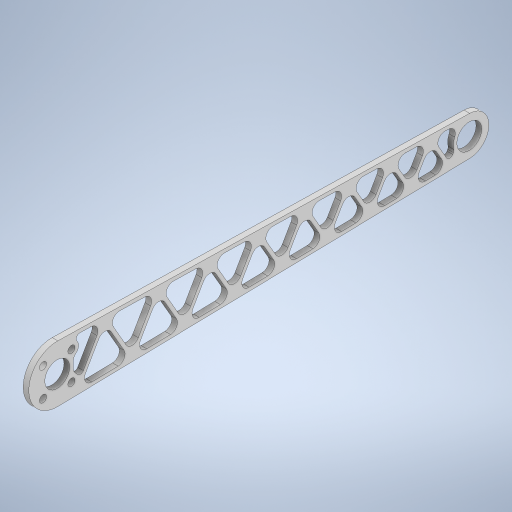
# Autodesk Inventor part: arm
Saved by Autodesk Inventor 2023 (Build 270158000, 158)
## iProperties
Created: 2022-09-10
Part Number: arm
Material: Generic
Document SubType Name: Modeling
Designer: deli
Density: 1 g/cm^3
Appearance: Default
Mass: 20.635 g
Surface Area: 151.802 cm^2
Volume: 20.635 cm^3
Author: deli
Autodesk Inventor part; units mm, degrees
ref_plane "YZ Plane" through (0, 0, 0) normal (1, 0, 0) x (0, 1, 0)
ref_plane "XZ Plane" through (0, 0, 0) normal (0, 1, 0) x (-1, 0, 0)
ref_plane "XY Plane" through (0, 0, 0) normal (0, 0, 1) x (1, 0, 0)
sketch "Sketch1" plane through (0, 0, 0) normal (1, 0, 0) x (0, 1, 0)
  circle A0 centre (62.068154, -4.109119) radius 2
  circle A1 centre (62.068154, -20.109119) radius 2
  circle A2 centre (46.068154, -20.109119) radius 2
  circle A3 centre (46.068154, -4.109119) radius 2
  line L0 (62.068154, -4.109119) -> (62.068154, -20.109119) construction
  line L1 (62.068154, -20.109119) -> (46.068154, -20.109119) construction
  line L2 (46.068154, -20.109119) -> (46.068154, -4.109119) construction
  line L3 (46.068154, -4.109119) -> (62.068154, -4.109119) construction
  circle A4 centre (54.068154, -12.109119) radius 7
  line L4 (62.068154, -4.109119) -> (46.068154, -20.109119) construction
  line L5 (62.068154, -20.109119) -> (46.068154, -4.109119) construction
  arc A5 (70.064438, -12.453946) -> (38.071871, -12.453946) centre (54.068154, -12.109119) ccw
  circle A6 centre (54.068154, -244.109119) radius 7
  line L6 (54.068154, -12.109119) -> (54.068154, -244.109119) construction
  arc A7 (43.070709, -244.346188) -> (65.065599, -244.346188) centre (54.068154, -244.109119) ccw
  line L7 (70.064438, -12.453946) -> (65.065599, -244.346188)
  line L8 (43.070709, -244.346188) -> (38.071871, -12.453946)
  line L9 (46.068154, -20.109119) -> (40.450729, -23.352341) construction
  line L10 (40.450729, -23.352341) -> (67.492484, -38.964905) construction
  line L11 (67.492484, -38.964905) -> (40.97387, -54.275434) construction
  line L12 (40.97387, -54.275434) -> (66.840508, -69.209545) construction
  line L13 (66.840508, -69.209545) -> (41.609816, -83.776492) construction
  line L14 (41.609816, -83.776492) -> (66.220197, -97.985302) construction
  line L15 (42.214877, -111.84478) -> (66.220197, -97.985302) construction
  line L16 (42.214877, -111.84478) -> (65.630012, -125.363515) construction
  line L17 (65.630012, -125.363515) -> (42.790551, -138.549883) construction
  line L18 (42.790551, -138.549883) -> (65.068491, -151.412058) construction
  line L19 (65.068491, -151.412058) -> (43.338268, -163.958008) construction
  line L20 (43.338268, -163.958008) -> (64.534241, -176.195509) construction
  line L21 (64.534241, -176.195509) -> (43.859383, -188.132144) construction
  line L22 (43.859383, -188.132144) -> (64.025937, -199.775309) construction
  line L23 (64.025937, -199.775309) -> (44.355189, -211.132221) construction
  line L24 (44.355189, -211.132221) -> (63.54232, -222.209916) construction
  line L25 (63.54232, -222.209916) -> (44.826916, -233.01526) construction
  line L26 (44.826916, -233.01526) -> (50.027004, -236.017532) construction
  line L27 (44.802331, -231.874754) -> (61.54232, -222.209916)
  line L28 (61.54232, -222.209916) -> (44.380395, -212.301473)
  line L29 (44.330604, -209.991715) -> (62.025937, -199.775309)
  line L30 (62.025937, -199.775309) -> (43.884588, -189.301396)
  line L31 (43.834797, -186.991637) -> (62.534241, -176.195509)
  line L32 (62.534241, -176.195509) -> (43.363473, -165.127261)
  line L33 (43.313682, -162.817502) -> (63.068491, -151.412058)
  line L34 (63.068491, -151.412058) -> (42.815757, -139.719136)
  line L35 (42.765966, -137.409377) -> (63.630012, -125.363515)
  line L36 (63.630012, -125.363515) -> (42.240082, -113.014033)
  line L37 (42.190291, -110.704274) -> (64.220197, -97.985302)
  line L38 (64.220197, -97.985302) -> (41.635021, -84.945744)
  line L39 (41.585231, -82.635985) -> (64.840508, -69.209545)
  line L40 (64.840508, -69.209545) -> (40.999075, -55.444687)
  line L41 (40.949284, -53.134928) -> (65.492484, -38.964905)
  line L42 (65.492484, -38.964905) -> (40.330666, -24.437723)
  line L43 (50.511319, -235.142451) -> (49.826916, -234.747311)
  line L44 (49.826916, -231.283209) -> (63.517115, -223.379169)
  line L45 (63.566906, -221.06941) -> (46.355189, -211.132221)
  line L46 (46.355189, -211.132221) -> (64.000732, -200.944562)
  line L47 (64.050523, -198.634803) -> (45.859383, -188.132144)
  line L48 (45.859383, -188.132144) -> (64.509035, -177.364762)
  line L49 (64.558826, -175.055003) -> (45.338268, -163.958008)
  line L50 (45.338268, -163.958008) -> (65.043286, -152.581311)
  line L51 (65.093076, -150.271552) -> (44.790551, -138.549883)
  line L52 (44.790551, -138.549883) -> (65.604807, -126.532767)
  line L53 (65.654598, -124.223009) -> (44.214877, -111.84478)
  line L54 (44.214877, -111.84478) -> (66.194992, -99.154554)
  line L55 (66.244783, -96.844796) -> (43.609816, -83.776492)
  line L56 (43.609816, -83.776492) -> (66.815303, -70.378797)
  line L57 (66.865094, -68.069039) -> (42.97387, -54.275434)
  line L58 (42.97387, -54.275434) -> (67.467279, -40.134158)
  line L59 (67.517069, -37.824399) -> (48.435104, -26.807421)
  arc A8 (48.312787, -23.419953) -> (49.941138, -21.109119) centre (46.068154, -20.109119) ccw
  arc A9 (63.066064, -244.303084) -> (51.976198, -235.355621) centre (54.068154, -244.109119) ccw
  arc A10 (67.796689, -24.853051) -> (64.554735, -23.242658) centre (65.797154, -24.809948) ccw
  line L60 (63.066064, -244.303084) -> (67.796689, -24.853051)
  arc A11 (58.194893, -21.109119) -> (64.554735, -23.242658) centre (62.068154, -20.109119) ccw
  line L61 (58.194893, -21.109119) -> (49.941138, -21.109119)
  line L62 (40.330666, -24.437723) -> (44.854331, -234.286992)
  arc A12 (48.312787, -23.419953) -> (48.435104, -26.807421) centre (49.435104, -25.07537) ccw
  arc A13 (49.826916, -231.283209) -> (49.826916, -234.747311) centre (50.826916, -233.01526) ccw
  arc A14 (50.511319, -235.142451) -> (51.976198, -235.355621) centre (51.511319, -233.4104) ccw
  point P0 (0, 0)
  dimension "d0" = 4
  dimension "d1" = 4
  dimension "d2" = 4
  dimension "d3" = 4
  dimension "d4" = 16
  dimension "d5" = 16
  dimension "d6" = 14
  dimension "d7" = 32
  dimension "d8" = 14
  dimension "d9" = 232
  dimension "d10" = 4
  dimension "d29" = 120
  dimension "d30" = 60
  dimension "d31" = 60
  dimension "d33" = 1
  dimension "d34" = 1
  dimension "d35" = 4
  dimension "d37" = 1
  dimension "d40" = 4
  dimension "d41" = 2
  dimension "d44" = 4
  dimension "d45" = 4
  dimension "d46" = 1
  dimension "d48" = 1
  dimension "d49" = 1
  dimension "d50" = 1
  dimension "d51" = 1
  dimension "d52" = 1
  dimension "d53" = 1
  dimension "d54" = 1
  dimension "d55" = 1
  dimension "d56" = 1
  dimension "d57" = 1
  dimension "d58" = 1
  dimension "d59" = 1
  dimension "d60" = 1
  dimension "d61" = 1
  dimension "d62" = 1
  dimension "d63" = 1
  dimension "d64" = 1
  dimension "d65" = 1
  dimension "d66" = 1
  dimension "d67" = 1
  dimension "d68" = 1
  dimension "d69" = 1
  dimension "d70" = 1
  dimension "d71" = 1
  dimension "d72" = 1
  dimension "d73" = 1
  dimension "d74" = 1
  dimension "d75" = 1
  dimension "d76" = 1
  dimension "d77" = 1
  dimension "d79" = 2
  dimension "d80" = 2
  constraints: 122 end point, 46 parallel, 18 point on circle, 15 centre point, 10 tangent, 3 coincident, 3 perpendicular, 2 vertical, 1 horizontal, 1 midpoint, 57 other
  measures "d0" diameter of A0
  measures "d1" diameter of A3
  measures "d2" diameter of A2
  measures "d3" diameter of A1
  measures "d4" distance of L0.start L0.end
  measures "d5" distance of L2.end L0.start
  measures "d6" diameter of A4
  measures "d7" diameter of A5
  measures "d8" diameter of A6
  measures "d9" distance of L6.start L6.end
  measures "d10" radial gap between concentric circles of A7 A6
  measures "d29" angle of L2 L9
  measures "d30" angle of L10 L9
  measures "d31" angle of L11 L10
  measures "d33" distance between parallel lines of L10 L42
  measures "d34" distance between parallel lines of L10 L59
  measures "d35" diameter of A10
  measures "d37" distance between parallel lines of L61 L1
  measures "d40" diameter of A12
  measures "d41" radial gap between concentric circles of A2 A8
  measures "d44" diameter of A13
  measures "d45" diameter of A14
  measures "d46" distance between parallel lines of L26 L43
  measures "d48" distance between parallel lines of L27 L25
  measures "d49" distance between parallel lines of L44 L25
  measures "d50" distance between parallel lines of L24 L45
  measures "d51" distance between parallel lines of L28 L24
  measures "d52" distance between parallel lines of L23 L46
  measures "d53" distance between parallel lines of L23 L29
  measures "d54" distance between parallel lines of L22 L47
  measures "d55" distance between parallel lines of L30 L22
  measures "d56" distance between parallel lines of L48 L21
  measures "d57" distance between parallel lines of L21 L31
  measures "d58" distance between parallel lines of L20 L49
  measures "d59" distance between parallel lines of L32 L20
  measures "d60" distance between parallel lines of L50 L19
  measures "d61" distance between parallel lines of L19 L33
  measures "d62" distance between parallel lines of L34 L18
  measures "d63" distance between parallel lines of L18 L51
  measures "d64" distance between parallel lines of L52 L17
  measures "d65" distance between parallel lines of L17 L35
  measures "d66" distance between parallel lines of L36 L16
  measures "d67" distance between parallel lines of L16 L53
  measures "d68" distance between parallel lines of L54 L15
  measures "d69" distance between parallel lines of L15 L37
  measures "d70" distance between parallel lines of L38 L14
  measures "d71" distance between parallel lines of L14 L55
  measures "d72" distance between parallel lines of L56 L13
  measures "d73" distance between parallel lines of L13 L39
  measures "d74" distance between parallel lines of L40 L12
  measures "d75" distance between parallel lines of L12 L57
  measures "d76" distance between parallel lines of L11 L58
  measures "d77" distance between parallel lines of L11 L41
extrude "Extrusion1" add sketch "Sketch1" along normal blind 3.175
fillet "Fillet1" radius 4 50 edges at (1.5875, 49.9411, -21.1091) (1.5875, 67.5171, -37.8244) (1.5875, 65.4925, -38.9649) (1.5875, 67.4673, -40.1342) (1.5875, 42.9739, -54.2754) (1.5875, 40.9493, -53.1349) (1.5875, 40.3307, -24.4377) (1.5875, 58.1949, -21.1091) (1.5875, 66.8651, -68.069) (1.5875, 66.8153, -70.3788) (1.5875, 64.8405, -69.2095) (1.5875, 40.9991, -55.4447) (1.5875, 41.5852, -82.636) (1.5875, 43.6098, -83.7765) (1.5875, 41.635, -84.9457) (1.5875, 66.2448, -96.8448) (1.5875, 64.2202, -97.9853) (1.5875, 66.195, -99.1546) (1.5875, 42.1903, -110.7043) (1.5875, 44.2149, -111.8448) (1.5875, 42.2401, -113.014) (1.5875, 63.63, -125.3635) (1.5875, 65.6546, -124.223) (1.5875, 65.6048, -126.5328) (1.5875, 42.766, -137.4094) (1.5875, 44.7906, -138.5499) (1.5875, 42.8158, -139.7191) (1.5875, 65.0931, -150.2716) (1.5875, 63.0685, -151.4121) (1.5875, 65.0433, -152.5813) (1.5875, 43.3137, -162.8175) (1.5875, 43.3635, -165.1273) (1.5875, 45.3383, -163.958) (1.5875, 64.5588, -175.055) (1.5875, 62.5342, -176.1955) (1.5875, 64.509, -177.3648) (1.5875, 43.8348, -186.9916) (1.5875, 45.8594, -188.1321) (1.5875, 43.8846, -189.3014) (1.5875, 64.0505, -198.6348) (1.5875, 62.0259, -199.7753) (1.5875, 64.0007, -200.9446) (1.5875, 44.3306, -209.9917) (1.5875, 44.3804, -212.3015) (1.5875, 46.3552, -211.1322) (1.5875, 63.5669, -221.0694) (1.5875, 61.5423, -222.2099) (1.5875, 63.5171, -223.3792) (1.5875, 44.8023, -231.8748) (1.5875, 63.0661, -244.3031)
equation "\"d1\" = d0"
equation "\"d2\" = d0"
equation "\"d3\" = d0"
equation "\"d31\" = d30"
body "Solid1"
